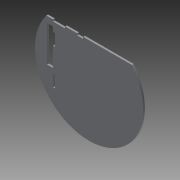
# Autodesk Inventor part: Base Plate
Saved by Autodesk Inventor 2015 (Build 190159000, 159)
## iProperties
Created: 2014-11-10
Part Number: Base Plate
Material: Generic
Document SubType Name: Modeling
Designer: karl
Density: 1 g/cm^3
Appearance: Default
Author: karl
Autodesk Inventor part; units mm, degrees
ref_plane "YZ Plane" through (0, 0, 0) normal (1, 0, 0) x (0, 1, 0)
ref_plane "XZ Plane" through (0, 0, 0) normal (0, 1, 0) x (-1, 0, 0)
ref_plane "XY Plane" through (0, 0, 0) normal (0, 0, 1) x (1, 0, 0)
sketch "Sketch1" plane through (0, 0, 0) normal (0, 1, 0) x (-1, 0, 0)
  circle A0 centre (0, 0) radius 90
  line L0 (-71.239, 55) -> (71.239, 55)
  dimension "d0" = 180
  dimension "d1" = 55
  constraints: 2 end point, 2 point on circle, 1 centre point, 1 coincident, 1 horizontal
  measures "d0" diameter of A0
  measures "d1" distance from line of point (0, 0) L0
extrude "Extrusion1" add sketch "Sketch1" along normal blind 3 contours A0 L0 picked at (-1.0947, 6.6866)
sketch "Sketch2" plane through (0, 3, 0) normal (0, 1, 0) x (1, 0, 0)
  line L0 (-70, -45) -> (-60, -45)
  line L1 (-60, -45) -> (-60, 15)
  line L2 (-60, 15) -> (-70, 15)
  line L3 (-70, 15) -> (-70, -45)
  line L4 (-70, -45) -> (-60, 15) construction
  line L5 (-60, -45) -> (-70, 15) construction
  point P0 (0, 0)
  point P1 (-65, -15)
  dimension "d4" = 10
  dimension "d5" = 60
  dimension "d6" = 15
  dimension "d7" = 65
  constraints: 12 end point, 2 midpoint, 2 parallel, 1 horizontal, 1 perpendicular
  measures "d4" distance of L2.end L1.end
  measures "d5" distance of L1.end L0.end
  measures "d6" vertical distance of point (0, 0) point (-65, -15)
  measures "d7" horizontal distance of point (0, 0) point (-65, -15)
extrude "Extrusion2" cut sketch "Sketch2" against normal blind 3
sketch "Sketch3" plane through (0, 3, 0) normal (0, 1, 0) x (1, 0, 0)
  line L0 (-71.239, -55) -> (71.239, -55) projected
  line L1 (-60, -55) -> (-40, -55)
  line L2 (-40, -55) -> (-40, -52)
  line L3 (-40, -52) -> (-60, -52)
  line L4 (-60, -52) -> (-60, -55)
  line L5 (-20, -55) -> (-10, -55)
  line L6 (-10, -55) -> (-10, -52)
  line L7 (-10, -52) -> (-20, -52)
  line L8 (-20, -52) -> (-20, -55)
  point P0 (0, 0)
  dimension "d10" = 20
  dimension "d11" = 3
  dimension "d12" = 10
  dimension "d13" = 3
  dimension "d14" = 10
  dimension "d15" = 20
  constraints: 16 end point, 4 parallel, 2 horizontal, 2 perpendicular, 2 point on line
  measures "d10" distance of L3.end L2.end
  measures "d11" distance of L2.end L1.end
  measures "d12" distance of L7.end L6.end
  measures "d13" distance of L6.end L5.end
  measures "d14" distance from line of point (0, 0) L6
  measures "d15" distance between parallel lines of L8 L2
extrude "Extrusion3" cut sketch "Sketch3" against normal blind 3
sketch "Sketch4" plane through (0, 3, 0) normal (0, 1, 0) x (1, 0, 0)
  line L0 (-60, -45) -> (-60, 15) projected
  line L1 (-60, -37) -> (-57, -37)
  line L2 (-57, -37) -> (-57, -17)
  line L3 (-57, -17) -> (-60, -17)
  line L4 (-60, -17) -> (-60, -37)
  line L5 (-57, 43) -> (-60, 43)
  line L6 (-60, 43) -> (-60, 23)
  line L7 (-60, 23) -> (-57, 23)
  line L8 (-57, 23) -> (-57, 43)
  line L9 (-60, -52) -> (-40, -52) projected
  point P0 (0, 0)
  dimension "d18" = 3
  dimension "d19" = 20
  dimension "d20" = 3
  dimension "d21" = 20
  dimension "d22" = 40
  dimension "d23" = 15
  constraints: 16 end point, 4 parallel, 2 horizontal, 2 perpendicular, 2 point on line
  measures "d18" distance of L3.end L2.end
  measures "d19" distance of L2.end L1.end
  measures "d20" distance of L7.end L6.end
  measures "d21" distance of L6.end L5.end
  measures "d22" distance between parallel lines of L3 L7
  measures "d23" distance between parallel lines of L9 L1
extrude "Extrusion4" cut sketch "Sketch4" against normal blind 3
sketch "Sketch5" plane through (0, 3, 0) normal (0, 1, 0) x (1, 0, 0)
  line L0 (31, 72.5) -> (-31, 72.5) construction
  line L1 (-31, 72.5) -> (-31, 37.5) construction
  line L2 (-31, 37.5) -> (31, 37.5) construction
  line L3 (31, 37.5) -> (31, 72.5) construction
  line L4 (31, 72.5) -> (-31, 37.5) construction
  line L5 (-31, 72.5) -> (31, 37.5) construction
  line L6 (-57, -37) -> (-57, -17) construction
  line L7 (-57, -21) -> (-31, -21) construction
  line L8 (-31, -21) -> (-31, -9) construction
  line L9 (-31, -9) -> (-57, -9) construction
  line L10 (-57, -9) -> (-57, -21) construction
  line L11 (-60, -45) -> (-70, -45) construction
  line L12 (-70, -45) -> (-70, 15) construction
  line L13 (-70, -15) -> (-60, -15) construction
  point P0 (0, 0)
  point P1 (0, 55)
  point P2 (0, 55)
  point P3 (-57, -15)
  point P4 (-65, -15)
  dimension "d26" = 62
  dimension "d27" = 35
  dimension "d28" = 55
  dimension "d29" = 26
  dimension "d30" = 12
  constraints: 22 end point, 6 midpoint, 4 parallel, 3 horizontal, 2 perpendicular, 1 horizontal alignment, 1 point on line, 1 vertical alignment
  measures "d26" distance of L2.end L1.end
  measures "d27" distance of L1.end L0.end
  measures "d28" distance of point (0, 0) point (0, 55)
  measures "d29" distance of L9.end L8.end
  measures "d30" distance of L8.end L7.end
sketch "Sketch6" plane through (0, 3, 0) normal (0, 1, 0) x (1, 0, 0)
  line L0 (-38, 63) -> (-35, 63)
  line L1 (-35, 63) -> (-35, 43)
  line L2 (-35, 43) -> (-38, 43)
  line L3 (-38, 43) -> (-38, 63)
  line L4 (-38, 3) -> (-35, 3)
  line L5 (-35, 3) -> (-35, 23)
  line L6 (-35, 23) -> (-38, 23)
  line L7 (-38, 23) -> (-38, 3)
  line L8 (-38, -37) -> (-35, -37)
  line L9 (-35, -37) -> (-35, -17)
  line L10 (-35, -17) -> (-38, -17)
  line L11 (-38, -17) -> (-38, -37)
  line L12 (-60, -52) -> (-40, -52) projected
  point P0 (0, 0)
  dimension "d32" = 3
  dimension "d33" = 20
  dimension "d34" = 35
  dimension "d35" = 3
  dimension "d36" = 20
  dimension "d37" = 20
  dimension "d38" = 3
  dimension "d39" = 20
  dimension "d40" = 20
  dimension "d41" = 15
  constraints: 24 end point, 6 parallel, 3 horizontal, 3 perpendicular, 2 collinear
  measures "d32" distance of L1.end L2.end
  measures "d33" distance of L0.end L1.end
  measures "d34" distance from line of point (0, 0) L1
  measures "d35" distance of L6.end L5.end
  measures "d36" distance of L5.end L4.end
  measures "d37" distance between parallel lines of L2 L6
  measures "d38" distance of L10.end L9.end
  measures "d39" distance of L9.end L8.end
  measures "d40" distance between parallel lines of L4 L10
  measures "d41" distance between parallel lines of L8 L12
extrude "Extrusion5" cut sketch "Sketch6" against normal blind 3
equation "\"d40\" = d36"
body "Solid1"
